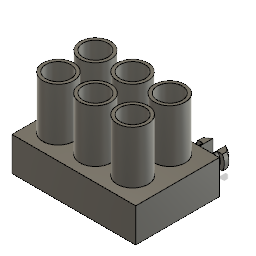
Pegboard_CNC_Holder_6mm Mill (Autodesk Fusion 360 design; units mm, degrees)
Autodesk Fusion 360 part; units mm, degrees
note: some values were not read from the file. Chosen so that the rebuilt part matches the saved one: which face or edge a step refers to; which pieces of a blend or face edit are solid.
sketch "Skizze1" plane through (0, 0, 0) normal (0, 1, 0) x (1, 0, 0)
  circle A0 centre (10, -15) radius 2.25
  dimension "d1" = 4.5
  measures "d1" diameter of A0
sketch "Skizze2" plane through (0, 0, 0) normal (0, 1, 0) x (1, 0, 0)
  circle A0 centre (5, -5) radius 1.75
  circle A1 centre (5, -5) radius 3
  dimension "d4" = 3.5
  dimension "d5" = 6
  measures "d4" diameter of A0
  measures "d5" diameter of A1
extrude "Extrusion3" add sketch "Skizze2" along normal blind 20 makes body 1
extrude "Extrusion2" add sketch "Skizze2" along normal blind 3 separate body contours A0 makes body 2
copy_body "Körper kopieren/einfügen1" bodies 1 2 makes body 3 makes body 4
move_body "Verschieben1" bodies 3 4 to x (1, 0, 0) y (0, 1, 0) z (0, 0, 1) at (8, 0, 0)
copy_body "Körper kopieren/einfügen2" bodies 3 4 makes body 5 makes body 6
move_body "Verschieben2" bodies 5 6 to x (1, 0, 0) y (0, 1, 0) z (0, 0, 1) at (8, 0, 0)
copy_body "Körper kopieren/einfügen3" bodies 5 6 makes body 7 makes body 8
move_body "Verschieben3" bodies 7 8 to x (1, 0, 0) y (0, 1, 0) z (0, 0, 1) at (8, 0, 0)
copy_body "Körper kopieren/einfügen4" bodies 7 8 makes body 9 makes body 10
move_body "Verschieben4" bodies 9 10 to x (1, 0, 0) y (0, 1, 0) z (0, 0, 1) at (8, 0, 0)
copy_body "Körper kopieren/einfügen5" bodies 9 10 8 7 6 5 4 1 2 3 makes body 11 makes body 12 makes body 13 makes body 14 makes body 15 makes body 16 makes body 17 makes body 18 makes body 19 makes body 20
move_body "Verschieben5" bodies 11 12 13 14 15 16 17 18 19 20 to x (1, 0, 0) y (0, 1, 0) z (0, 0, 1) at (0, 0, 8)
sketch "Skizze3" plane through (0, 0, 0) normal (0, 1, 0) x (1, 0, 0)
  line L0 (1, -1) -> (41, -1)
  line L1 (41, -1) -> (41, -17)
  line L2 (41, -17) -> (1, -17)
  line L3 (1, -17) -> (1, -1)
extrude "Extrusion4" add sketch "Skizze3" along normal blind 3 separate body makes body 21
extrude "Extrusion5" add 1 faces at (14.3333, 3, 6.3333) along direction (0, 1, 0) blind 7 on bodies 21 bodies 21 1 2 3 4 5 6 7 8 9 10 11 12 13 14 15 16 17 18 19 20
extrude "Extrusion6" cut 10 faces at (4.518, 10, 4.6714) (12.7083, 10, 5.5052) (20.6363, 10, 5.4561) (28.0468, 10, 4.3501) (36.4426, 10, 4.8281) (36.5609, 10, 12.0434) (29.4276, 10, 13.2604) (21.3637, 10, 13.4561) (5.5129, 10, 13.9398) (13.2278, 10, 13.3477) along direction (0, -1, 0) blind 8 on bodies 21 bodies 21
sketch "Skizze5" plane through (0, 0, 1) normal (0, 0, -1) x (-1, 0, 0)
  line L0 (-41, 0) -> (-1, 0)
  line L1 (-1, 0) -> (-1, 10)
  line L2 (-1, 10) -> (-41, 10)
  line L3 (-41, 10) -> (-41, 0)
  circle A0 centre (-33, 5) radius 3.3
  line L4 (-31.4904, 8.6612) -> (-34.5096, 8.6612)
  line L5 (-34.5096, 8.6612) -> (-34.5096, 1.3388)
  line L6 (-34.5096, 1.3388) -> (-31.4904, 1.3388)
  line L7 (-31.4904, 1.3388) -> (-31.4904, 8.6612)
  line L8 (-31.4904, 8.6612) -> (-34.5096, 1.3388) construction
  line L9 (-34.5096, 8.6612) -> (-31.4904, 1.3388) construction
  point P0 (-33, 5)
  dimension "d23" = 6.6
  measures "d23" diameter of A0
extrude "Extrusion7" add sketch "Skizze5" along normal blind 5 contours A0 L7 | A0 L5 L7 | A0 L5 bodies 21
sketch "Skizze6" plane through (0, 0, -4) normal (0, 0, -1) x (-1, 0, 0)
  circle A0 centre (-33, 5) radius 3.3
  circle A1 centre (-33, 5) radius 4.605
  dimension "d26" = 9.21
  measures "d26" diameter of A1
extrude "Extrusion8" add sketch "Skizze6" along normal blind 3 separate body makes body 22
split "Teilen1" by plane through (1, 0, 1) normal (0, 0, -1) bodies 21 makes body 23 at (29.7041, 5.1645, -0.6667)
extrude "Extrusion9" add 1 faces at (34.1, 6.72, -4) along direction (0, 0, -1) blind 3 on bodies 23 bodies 23 22
sketch "Skizze7" plane through (0, 0, -7) normal (0, 0, -1) x (-1, 0, 0)
  circle A0 centre (-33, 5) radius 4.605
  line L0 (-31, 10) -> (-35, 10)
  line L1 (-35, 10) -> (-35, 0)
  line L2 (-35, 0) -> (-31, 0)
  line L3 (-31, 0) -> (-31, 10)
  line L4 (-31, 10) -> (-35, 0) construction
  line L5 (-35, 10) -> (-31, 0) construction
  line L6 (-32, 10) -> (-26, 10)
  point P0 (-33, 5)
extrude "Extrusion10" cut sketch "Skizze7" against normal blind 8 contours A0 L1 L3 bodies 23 makes body 24 at (35, 5.875, -0.6667)
chamfer "Fase1" distance 1.5 angle 45 2 edges at (37.605, 5, -7) (28.395, 5, -7) on bodies 23 24
copy_body "Körper kopieren/einfügen6" bodies 24 23 makes body 25 makes body 26
move_body "Verschieben6" bodies 25 26 to x (1, 0, 0) y (0, 1, 0) z (0, 0, 1) at (-25, 0, 0)
delete_face "Fläche löschen1" 4 faces at (7.9851, 13.3333, 12.7013) (7.5656, 20, 13.236) (6.7413, 8, 12.8258) (5.5574, 2, 13.1719) on bodies 21
delete_face "Fläche löschen2" 4 faces at (7.9851, 13.3333, 4.7013) (7.5656, 20, 5.236) (6.7413, 8, 4.8258) (4.8702, 2, 4.4313) on bodies 21
delete_face "Fläche löschen3" 4 faces at (15.9851, 13.3333, 12.7013) (15.5656, 20, 13.236) (14.7413, 8, 12.8258) (12.8585, 2, 13.438) on bodies 21
delete_face "Fläche löschen4" 4 faces at (15.9851, 13.3333, 4.7013) (15.5656, 20, 5.236) (14.7413, 8, 4.8258) (13.0426, 2, 4.4313) on bodies 21
delete_face "Fläche löschen5" 4 faces at (23.9851, 13.3333, 12.7013) (23.5656, 20, 13.236) (22.7413, 8, 12.8258) (20.6889, 2, 12.4098) on bodies 21
delete_face "Fläche löschen6" 4 faces at (23.9851, 13.3333, 4.7013) (23.5656, 20, 5.236) (22.7413, 8, 4.8258) (20.8702, 2, 4.4313) on bodies 21
delete_face "Fläche löschen7" 4 faces at (31.9851, 13.3333, 12.7013) (31.5656, 20, 13.236) (30.7413, 8, 12.8258) (28.6889, 2, 12.4098) on bodies 21
delete_face "Fläche löschen8" 4 faces at (31.9851, 13.3333, 4.7013) (31.5656, 20, 5.236) (30.7413, 8, 4.8258) (28.8702, 2, 4.4313) on bodies 21
delete_face "Fläche löschen9" 4 faces at (39.9851, 13.3333, 12.7013) (39.5656, 20, 13.236) (36.526, 8, 11.3154) (37.4276, 2, 12.2594) on bodies 21
delete_face "Fläche löschen10" 4 faces at (39.9851, 13.3333, 4.7013) (39.5656, 20, 5.236) (35.842, 8, 3.6879) (36.4426, 2, 4.8281) on bodies 21
sketch "Skizze8" plane through (0, 0, -7) normal (0, 0, -1) x (-1, 0, 0)
  arc A0 (-35, 7.3751) -> (-35, 2.6249) centre (-33, 5) ccw
  line L0 (-35, 2.6249) -> (-35, 7.3751)
  line L1 (-35, 7.3751) -> (-1, 7.3751)
  line L2 (-1, 7.3751) -> (-1, 10)
  line L3 (-1, 10) -> (-35, 10)
  line L4 (-35, 10) -> (-35, 7.3751)
  line L5 (-6, 7.3751) -> (-41, 7.3751)
  line L6 (-41, 7.3751) -> (-41, 10)
  line L7 (-41, 10) -> (-6, 10)
  line L8 (-6, 10) -> (-6, 7.3751)
  point P0 (-1, 10)
  point P1 (-6, 7.3751)
  point P2 (-41, 10)
extrude "Extrusion11" cut sketch "Skizze8" against normal blind 8 contours L1 L3 L4 L5 L7 L8 | L4 L5 L6 L7 | L1 L2 L3 L8 bodies 23 24 25 26
sketch "Skizze9" plane through (0, 0, -7) normal (0, 0, -1) x (-1, 0, 0)
  arc A0 (-10, 7.3751) -> (-10, 2.6249) centre (-8, 5) ccw
  line L0 (-10, 2.6249) -> (-10, 7.3751)
  line L1 (-1, 0) -> (-35, 0)
  line L2 (-35, 0) -> (-35, 2.6249)
  line L3 (-35, 2.6249) -> (-1, 2.6249)
  line L4 (-1, 2.6249) -> (-1, 0)
  line L5 (-41, 0) -> (-6, 0)
  line L6 (-6, 0) -> (-6, 2.6249)
  line L7 (-6, 2.6249) -> (-41, 2.6249)
  line L8 (-41, 2.6249) -> (-41, 0)
  point P0 (-1, 0)
  point P1 (-35, 2.6249)
  point P2 (-41, 0)
  point P3 (-6, 2.6249)
extrude "Extrusion12" cut sketch "Skizze9" against normal blind 8 contours L1 L2 L3 L5 L6 L7 | L2 L5 L7 L8 | L1 L3 L4 L6 bodies 23 24 25 26
extrude "Extrusion13" add 1 faces at (27.6667, 6.6667, 17) along direction (0, 0, 1) blind 19 on bodies 21 bodies 21
sketch "Skizze10" plane through (0, 10, 0) normal (0, 1, 0) x (-1, 0, 0)
  line L0 (-41, 36) -> (-41, 1)
  line L1 (-41, 1) -> (-1, 1)
  line L2 (-1, 1) -> (-1, 36)
  line L3 (-1, 36) -> (-41, 36)
  circle A0 centre (-8, 8) radius 4
  circle A1 centre (-8, 8) radius 5
  dimension "d45" = 8
  dimension "d46" = 10
  measures "d45" diameter of A0
  measures "d46" diameter of A1
extrude "Extrusion14" cut sketch "Skizze10" against normal blind 2 contours L0 L1 L2 L3 bodies 21
extrude "Extrusion15" cut 1 faces at (27.6667, 0, 12.6667) along direction (0, 1, 0) blind 2 on bodies 21 bodies 21
delete_face "Fläche löschen11" 1 faces at (3.0248, 9.3333, 7.5022) on bodies 21
sketch "Skizze11" plane through (0, 8, 0) normal (0, 1, 0) x (-1, 0, 0)
  line L0 (-1, 36) -> (-41, 36)
  line L1 (-41, 36) -> (-41, 1)
  line L2 (-41, 1) -> (-1, 1)
  line L3 (-1, 1) -> (-1, 36)
  circle A0 centre (-8, 8) radius 4
  circle A1 centre (-8, 8) radius 5
  dimension "d51" = 8
  dimension "d52" = 10
  measures "d51" diameter of A0
  measures "d52" diameter of A1
extrude "Extrusion16" add sketch "Skizze11" along normal blind 20 separate body contours A1 makes body 27
copy_body "Körper kopieren/einfügen7" bodies 27 makes body 28
move_body "Verschieben7" bodies 28 to x (1, 0, 0) y (0, 1, 0) z (0, 0, 1) at (12, 0, 0)
copy_body "Körper kopieren/einfügen8" bodies 28 makes body 29
move_body "Verschieben8" bodies 29 to x (1, 0, 0) y (0, 1, 0) z (0, 0, 1) at (12, 0, 0)
copy_body "Körper kopieren/einfügen9" bodies 27 28 29 makes body 30 makes body 31 makes body 32
move_body "Verschieben9" bodies 30 31 32 to x (1, 0, 0) y (0, 1, 0) z (0, 0, 1) at (0, 0, 12)
extrude "Extrusion17" cut 1 faces at (27.6667, 4, 36) along direction (0, 0, -1) blind 8 on bodies 21 bodies 21
extrude "Extrusion18" add 1 faces at (14.3333, 8, 10) along direction (0, 1, 0) blind 3 on bodies 21 bodies 21 27 28 29 30 31 32
extrude "Extrusion19" add 1 faces at (27.6667, 2, 10) along direction (0, -1, 0) blind 2 on bodies 21 bodies 21
extrude "Extrusion20" cut 6 faces at (8.6842, 11, 9.2709) (19.1687, 11, 6.1715) (32.9634, 11, 10.4546) (9.0541, 11, 21.2431) (21.0226, 11, 22.0616) (30.6667, 11, 18.1862) along direction (0, -1, 0) blind 9 on bodies 21 bodies 21
